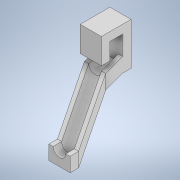
# Autodesk Inventor part: ramp(2)
Saved by Autodesk Inventor 2021 (Build 250183000, 183)
## iProperties
Created: 2021-03-29
Part Number: ramp(2)
Material: Generic
Document SubType Name: Modeling
Designer: jtri402
Density: 1 g/cm^3
Appearance: Default
Author: jtri402
Autodesk Inventor part; units mm, degrees
ref_plane "YZ Plane" through (0, 0, 0) normal (1, 0, 0) x (0, 1, 0)
ref_plane "XZ Plane" through (0, 0, 0) normal (0, 1, 0) x (-1, 0, 0)
sketch "Sketch5" plane through (0, 0, 0) normal (0, 0, 1) x (1, 0, 0)
  line L0 (-12.5, 10) -> (12.5, 10)
  line L1 (12.5, 10) -> (12.5, -40)
  line L2 (12.5, -40) -> (-12.5, -40)
  line L3 (-12.5, -40) -> (-12.5, 10)
  circle A0 centre (0, 0) radius 7.5
  dimension "d11" = 25
  dimension "d12" = 50
  dimension "d13" = 15
  dimension "d14" = 10
  dimension "d15" = 12.5
  constraints: 8 end point, 2 parallel, 1 centre point, 1 coincident, 1 horizontal, 1 perpendicular
  measures "d11" distance of L0.start L0.end
  measures "d12" distance of L0.end L1.end
  measures "d13" diameter of A0
  measures "d14" distance from line of point (0, 0) L0
  measures "d15" distance from line of point (0, 0) L1
extrude "Extrusion4" add sketch "Sketch5" along normal blind 10
sketch "Sketch6" plane through (0, 0, 10) normal (0, 0, 1) x (1, 0, 0)
  circle A0 centre (0, 0) radius 7.5 projected
  line L0 (-7.5, 0) -> (-12.5, 0)
  line L1 (-12.5, 10) -> (-12.5, -40) projected
  line L2 (-12.5, 10) -> (-12.5, 0)
  line L3 (12.5, 10) -> (-12.5, 10) projected
  line L4 (12.5, -40) -> (12.5, 10) projected
  line L5 (-12.5, 10) -> (12.5, 10)
  line L6 (12.5, 10) -> (12.5, 0)
  line L7 (12.5, 0) -> (7.5, 0)
  arc A1 (7.5, 0) -> (-7.5, 0) centre (0, 0) ccw
  constraints: 10 end point, 4 point on circle, 3 perpendicular, 2 horizontal, 1 centre point, 1 concentric, 1 point on line
extrude "Extrusion5" add sketch "Sketch6" along normal blind 15 contours A0 L0 L1 L3 L4 L7
sketch "Sketch7" plane through (0, 0, 25) normal (0, 0, 1) x (1, 0, 0)
  line L0 (-12.5, 10) -> (-12.5, -40) projected
  line L1 (12.5, -40) -> (12.5, 0) projected
  line L2 (-12.5, 10) -> (12.5, 10)
  line L3 (12.5, 10) -> (12.5, -20)
  line L4 (12.5, -20) -> (-12.5, -20)
  line L5 (-12.5, -20) -> (-12.5, 10)
  point P0 (0, 0)
  point P1 (-12.5, -20)
  point P2 (12.5, 0)
  dimension "d20" = 30
  constraints: 8 end point, 2 parallel, 1 horizontal, 1 midpoint, 1 perpendicular
  measures "d20" distance of L2.end L3.end
extrude "Extrusion6" add sketch "Sketch7" along normal blind 10
ref_plane "Work Plane1" through (0, -40, 0) normal (1, 0, 0) x (0, 0, -1)
ref_plane "Work Plane2" through (0, 0, 90) normal (0, 0, 1) x (1, 0, 0)
sketch "Sketch12" plane through (0, 0, 90) normal (0, 0, 1) x (1, 0, 0)
  line L0 (0, 28.6) -> (0, -101.6) projected
  line L1 (-23.1, 0) -> (51.1, 0) projected
  arc A0 (20.5, -66) -> (35.5, -66) centre (28, -66) ccw
  line L2 (20.5, -66) -> (15.5, -66)
  line L3 (15.5, -66) -> (15.5, -83)
  line L4 (15.5, -83) -> (40.5, -83)
  line L5 (40.5, -83) -> (40.5, -66)
  line L6 (40.5, -66) -> (35.5, -66)
  point P0 (0, 0)
  dimension "d55" = 15
  dimension "d56" = 5
  dimension "d57" = 17
  dimension "d58" = 25
  constraints: 10 end point, 3 perpendicular, 2 point on circle, 2 point on line, 1 centre point, 1 horizontal
  measures "d55" diameter of A0
  measures "d56" distance of L2.start L2.end
  measures "d57" distance of L2.end L3.end
  measures "d58" distance of L3.end L4.end
sketch "Sketch13" plane through (0, 0, 10) normal (0, 0, 1) x (1, 0, 0)
  line L0 (-7.5, -23) -> (-12.5, -23)
  line L1 (-12.5, 0) -> (-12.5, -40) projected
  line L2 (-12.5, -23) -> (-12.5, -40)
  line L3 (-12.5, -40) -> (12.5, -40) projected
  line L4 (-12.5, -40) -> (12.5, -40)
  line L5 (12.5, -40) -> (12.5, -23)
  line L6 (12.5, -40) -> (12.5, 0) projected
  line L7 (12.5, -23) -> (7.5, -23)
  arc A0 (-7.5, -23) -> (7.5, -23) centre (0, -23) ccw
  line L8 (-12.5, -31.5) -> (12.5, -31.5)
  point P0 (0, 0)
  dimension "d48" = 5
  dimension "d49" = 5
  dimension "d50" = 7.5
  dimension "d51" = 17
  constraints: 12 end point, 4 point on line, 2 collinear, 2 point on circle, 1 centre point, 1 horizontal, 1 midpoint, 1 perpendicular
  measures "d48" distance of L0.start L0.end
  measures "d49" distance of L5.end L7.end
  measures "d50" radius of A0
  measures "d51" distance between parallel lines of L3 L0
sketch "Sketch14" plane through (0, 0, 0) normal (1, 0, 0) x (0, 1, 0)
  line L0 (-40, 10) -> (0, 10) projected
  line L1 (-40, 0) -> (-40, 10) projected
  line L2 (-31.5, 10) -> (-38.7794, 30)
  point P0 (0, 0)
  dimension "d62" = 8.5
  dimension "d63" = 70
  dimension "d64" = 20
  constraints: 2 end point, 1 point on line
  measures "d62" distance of L0.start L2.start
  measures "d63" angle of L0 L2
  measures "d64" vertical distance of L0.start L2.end
sweep "Sweep2" add profiles "Sketch13" path "Sketch14" path curves L2
loft "Loft1" add profiles "Sketch12" section 1 edges at (0, -47.2794, 30) (12.5, -38.7794, 30) (10, -30.2794, 30) (0, -37.7794, 30) (-10, -30.2794, 30) (-12.5, -38.7794, 30)
sketch "Sketch15" plane through (15.5, -83, 90) normal (0, 0, 1) x (1, 0, 0)
  line L0 (5, 17) -> (-23, 52.7206) projected
  line L1 (0, 17) -> (5, 17) projected
  line L2 (5, 17) -> (0, 17)
  line L3 (0, 0) -> (0, 17) projected
  line L4 (0, 17) -> (0, 0)
  line L5 (25, 0) -> (0, 0) projected
  line L6 (0, 0) -> (25, 0)
  line L7 (25, 17) -> (25, 0) projected
  line L8 (25, 0) -> (25, 17)
  line L9 (20, 17) -> (25, 17) projected
  line L10 (25, 17) -> (20, 17)
  arc A0 (5, 17) -> (20, 17) centre (12.5, 17) ccw
  point P0 (-15.5, 83)
  constraints: 10 end point, 3 collinear, 2 point on circle, 1 centre point, 1 horizontal, 1 perpendicular
extrude "Extrusion7" add sketch "Sketch15" along normal blind 10
equation "\"d15\" = 0.5 * d11"
body "Solid2"
